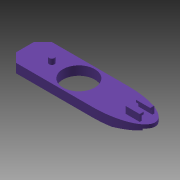
# Autodesk Inventor part: Guide
Saved by Autodesk Inventor 2015 (Build 190141000, 141)
## iProperties
Created: 2008-06-07
Part Number: Guide
Document SubType Name: Modeling
Designer: tangg
Density: 0.94 g/cm^3
Mass: 82.2056 g
Surface Area: 237.47 cm^2
Volume: 82.2056 cm^3
Stock Number: Guide
Material: UHMW, Black
Appearance: Violet
Author: tangg
Autodesk Inventor part; units mm, degrees
ref_plane "XZ Plane" through (0, 0, 0) normal (0, 1, 0) x (-1, 0, 0)
sketch "Sketch1" plane through (0, 0, 0) normal (0, 0, 1) x (1, 0, 0)
  line L0 (107.721093, 0) -> (-76.2, 0)
  line L1 (-76.2, 0) -> (-76.2, -12.7)
  line L2 (-76.2, -12.7) -> (69.621093, -12.700026)
  line L3 (107.721093, -6.350016) -> (107.721093, 0)
  line L4 (107.721093, -6.350016) -> (69.621093, -12.700026)
  point P0 (0, 0)
  dimension "d19" = 183.92109
  dimension "d20" = 76.2
  dimension "d21" = 12.7
  dimension "d22" = 38.1
  constraints: 10 end point, 1 point on line, 1 vertical
  measures "d19" distance of L0.start L0.end
  measures "d20" distance from line of point (0, 0) L1
  measures "d21" distance of L0.end L1.end
  measures "d22" horizontal distance of L3.start L2.end
extrude "Extrusion2" add sketch "Sketch1" along normal blind 25.4
sketch "Sketch2" plane through (-76.2, 0, 0) normal (0, 1, 0) x (1, 0, 0)
  circle A0 centre (76.2, 0) radius 22.5
  dimension "d25" = 45
  constraints: 1 centre point, 1 coincident
  measures "d25" diameter of A0
extrude "Extrusion3" cut sketch "Sketch2" against normal through all
mirror "Mirror1" about plane through (14.352169, -5.990033, 0) normal (0, 0, -1) of "Extrusion2", "Extrusion3"
sketch "Sketch4" plane through (-76.2, 0, 25.4) normal (0, 1, 0) x (1, 0, 0)
  circle A0 centre (38.1, 25.4) radius 3.81
  line L0 (-36.784219, 25.4) -> (220.705311, 25.4)
  point P0 (76.2, 25.4)
  dimension "d13" = 7.62
  dimension "d39" = 38.1
  constraints: 1 centre point, 1 point on line
  measures "d13" diameter of A0
  measures "d39" distance of A0.centre point (76.2, 25.4)
extrude "Extrusion5" add sketch "Sketch4" along normal blind 7.62
ref_plane "Work Plane1" through (76.2, 0, 0) normal (1, 0, 0) x (0, 1, 0)
sketch "Sketch10" plane through (69.621093, -12.700026, -25.4) normal (-0.0000002, -1, 0) x (1, -0.0000002, 0)
  line L0 (-69.621095, 36.62532) -> (38.099999, 36.62532)
  line L1 (-69.621095, 14.17468) -> (38.1, 14.17468)
  circle A0 centre (-69.621095, 25.4) radius 11.22532
  line L2 (-69.621095, 36.62532) -> (-69.621095, 14.17468) construction
  line L3 (38.099999, 0) -> (38.099999, 50.8) construction
  line L4 (38.099999, 36.62532) -> (38.1, 14.17468)
  point P0 (-69.621095, 25.4)
  constraints: 8 end point, 4 point on circle, 3 point on line, 1 centre point, 1 horizontal
extrude "Extrusion11" cut sketch "Sketch10" against normal mid plane 15.24
ref_plane "Work Plane4" through (63.5, 0, 0) normal (1, 0, 0) x (0, 1, 0)
sketch "Sketch5" plane through (76.2, 0, 0) normal (1, 0, 0) x (0, 1, 0)
  line L0 (-1.5875, -10.237854) -> (9.525, -10.237854)
  line L1 (9.525, -10.237854) -> (9.525, 10.237854)
  line L2 (9.525, 10.237854) -> (-1.5875, 10.237854)
  line L3 (-1.5875, 10.237854) -> (-1.5875, -10.237854)
  line L4 (9.525, -7.62) -> (0, -7.62)
  line L5 (0, -7.62) -> (0, 7.62)
  line L6 (0, 7.62) -> (9.525, 7.62)
  line L7 (9.525, 7.62) -> (9.525, -7.62)
  line L8 (0, 25.4) -> (0, -25.4)
  line L9 (9.525, -7.62) -> (6.5, -7.62)
  line L10 (6.5, -7.62) -> (6.5, -4.62)
  line L11 (6.5, -4.62) -> (9.525, -4.62)
  line L12 (9.525, -4.62) -> (9.525, -7.62)
  line L13 (9.525, 7.62) -> (6.5, 7.62)
  line L14 (6.5, 7.62) -> (6.5, 4.62)
  line L15 (6.5, 4.62) -> (9.525, 4.62)
  line L16 (9.525, 4.62) -> (9.525, 7.62)
  point P0 (0, 0)
  point P1 (0, 0)
  point P2 (9.525, 0)
  dimension "d14" = 15.24
  dimension "d50" = 6.5
  dimension "d51" = 3
  dimension "d52" = 3
  constraints: 32 end point, 3 midpoint, 1 collinear, 1 horizontal alignment, 1 point on line
  measures "d14" distance between parallel lines of L6 L4
  measures "d50" distance between parallel lines of L5 L10
  measures "d51" distance between parallel lines of L9 L11
  measures "d52" distance between parallel lines of L6 L15
extrude "Extrusion6" add sketch "Sketch5" along normal blind 20 contours L3 L2 L8 L5 L0 | L8 L4 L1 L0 | L2 L1 L6 L8 | L4 L10 L11 L1 | L6 L1 L15 L14
fillet "Fillet1" radius 0.635 4 edges at (96.2, 9.525, 7.4289) (76.2, 9.525, 7.4289) (76.2, 9.525, -7.4289) (96.2, 9.525, -7.4289)
chamfer "Chamfer1" distance 12.7 angle 45 2 edges at (-76.2, -6.35, -25.4) (-76.2, -6.35, 25.4)
sketch "Sketch11" plane through (63.5, 0, 0) normal (1, 0, 0) x (0, 1, 0)
  line L0 (-5.080017, 11.22532) -> (-12.700026, 11.22532)
  ellipse E0 centre (-5.080014, 0) end of major axis (-5.080014, -22.5) minor radius 0.000004 (-5.080017, 11.22532) -> (-5.080017, -11.22532) ccw
  line L1 (-12.700026, -11.22532) -> (-5.080017, -11.22532)
  line L2 (-12.700026, 11.22532) -> (-6.350016, 11.22532)
  line L3 (-6.350016, 11.22532) -> (-5.080033, 11.22532)
  line L4 (-5.080033, 11.22532) -> (-5.080033, -11.22532)
  line L5 (-6.350016, -11.22532) -> (-12.700026, -11.22532)
  arc A0 (-12.700026, 11.22532) -> (-12.700026, -11.22532) centre (-10.847911, 0) ccw
  circle A1 centre (-15.875014, 0) radius 2.54
  ellipse E1 centre (-12.700014, 0) end of major axis (-12.700014, 22.5) minor radius 0.000004 (-12.700026, -11.22532) -> (-12.700026, 11.22532) ccw
  point P0 (0, 0)
  dimension "d48" = 3.175
  dimension "d49" = 5.08
  constraints: 2 centre point, 2 point on circle, 2 other
  measures "d48" distance of point (-12.7, 0) A1.centre
  measures "d49" diameter of A1
extrude "Extrusion12" add sketch "Sketch11" along normal mid plane 12.7
sketch "Sketch12" plane through (107.721093, 0, 25.4) normal (0, 1, 0) x (1, 0, 0)
  line L0 (-171.221093, 50.8) -> (0, 50.8)
  line L1 (0, 0) -> (0, 50.8)
  line L2 (-171.221093, 0) -> (0, 0)
  line L3 (0, 25.4) -> (-107.721093, 25.4) construction
  ellipse E0 centre (-63.5, 25.4) end of major axis (0, 25.4) minor radius 25.4 (-63.5, 0) -> (-63.5, 50.8) ccw
  constraints: 3 point on line, 2 end point, 1 midpoint, 5 other
extrude "Extrusion13" cut sketch "Sketch12" against normal through all
body "Solid1"
